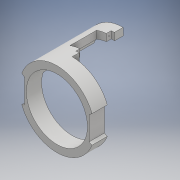
# Autodesk Inventor part: X-axis-gimbal-part
Saved by Autodesk Inventor 2017 (Build 210142000, 142)
## iProperties
Part Number: X-axis-gimbal-part
Material: 常规
Document SubType Name: Modeling
Designer: Lenovo
Density: 1 g/cm^3
Appearance: 默认
Author: Lenovo
Autodesk Inventor part; units mm, degrees
ref_plane "YZ Plane" through (0, 0, 0) normal (1, 0, 0) x (0, 1, 0)
ref_plane "XZ Plane" through (0, 0, 0) normal (0, 1, 0) x (-1, 0, 0)
sketch "Sketch1" plane through (0, 0, 0) normal (0, 1, 0) x (-1, 0, 0)
  circle A0 centre (0, 0) radius 37.0055
  circle A1 centre (0, 0) radius 29.8875
  constraints: 2 centre point, 2 coincident
extrude "Extrusion1" add sketch "Sketch1" along normal blind 15 contours A0 | A1
sketch "Sketch2" plane through (0, 15, 0) normal (0, 1, 0) x (1, 0, 0)
  circle A0 centre (0, 0) radius 37.0055 projected
  circle A1 centre (0, 0) radius 30.0306
  constraints: 1 centre point, 1 coincident
extrude "Extrusion2" cut sketch "Sketch2" against normal blind 15 contours A1
sketch "Sketch3" plane through (0, 15, 0) normal (0, 1, 0) x (1, 0, 0)
  circle A0 centre (0, 0) radius 37.0055 projected
  line L0 (-34.4949, -13.3982) -> (-31.6379, -11.0586)
  line L1 (-31.6379, -11.0586) -> (-31.6379, 12.0839)
  line L2 (-31.6379, 12.0839) -> (-34.4949, 13.3982)
  constraints: 6 end point, 2 point on circle, 1 vertical
extrude "Extrusion3" cut sketch "Sketch3" against normal blind 15 contours L2 L1 L0 A0 picked at (-33.4271, 0.3418)
sketch "Sketch4" plane through (0, 15, 0) normal (0, 1, 0) x (1, 0, 0)
  arc A0 (-34.4949, -13.3982) -> (-34.4949, 13.3982) centre (0, 0) ccw projected
  line L0 (-31.6379, -11.0586) -> (-31.6379, 12.0839) projected
  line L1 (31.575, 12.0839) -> (31.575, -11.0586)
  line L2 (31.575, -11.0586) -> (34.4949, -13.3982)
  line L3 (31.575, 12.0839) -> (34.4949, 13.3982)
  constraints: 6 end point, 2 point on circle
extrude "Extrusion4" cut sketch "Sketch4" against normal blind 15
sketch "Sketch5" plane through (0, 15, 0) normal (0, 1, 0) x (1, 0, 0)
  circle A0 centre (0, 0) radius 30.0306 projected
  line L0 (-31.6379, -11.0586) -> (-34.4949, -13.3982) projected
  arc A1 (-34.4949, -13.3982) -> (34.4949, -13.3982) centre (0, 0) ccw projected
  line L1 (-31.6379, -11.0586) -> (-31.6379, 12.0839) projected
  circle A2 centre (0, 0) radius 30.0306 projected
  line L2 (-31.6379, -11.0586) -> (-28.482, -9.519)
  line L3 (0, -37.0055) -> (0.2981, -30.0291)
  constraints: 5 point on circle, 4 end point
extrude "Extrusion5" add sketch "Sketch5" along normal blind 50 contours A0 L3 A1 L0 L2
ref_plane "Work Plane1" through (0, 15, 37.0055) normal (0, 0, 1) x (1, 0, 0)
sketch "Sketch6" plane through (0, 15, 37.0055) normal (0, 0, 1) x (1, 0, 0)
  line L0 (0.2981, 0) -> (0.2981, 50) projected
  line L1 (0.2981, 41.3903) -> (-3.1652, 41.3903)
  line L2 (-3.1652, 41.3903) -> (-3.1652, 36.7258)
  line L3 (-3.1652, 36.7258) -> (-12.8273, 36.7258)
  line L4 (-12.8273, 36.7258) -> (-12.8273, 10.738)
  line L5 (-12.8273, 10.738) -> (-3.1652, 10.738)
  line L6 (-3.1652, 10.738) -> (-3.1652, 6.7398)
  line L7 (-3.1652, 6.7398) -> (0.2981, 6.7398)
  point P0 (0, -15)
  constraints: 14 end point, 5 perpendicular, 2 horizontal, 2 point on line
extrude "Extrusion6" cut sketch "Sketch6" against normal blind 10
hole "Hole1" at (-3.1652, 23.7389, 33.3666) direction (-1, 0, 0) diameter 1 depth 3 tip angle 118
hole "Hole2" at (-3.1652, 54.058, 33.3666) direction (-1, 0, 0) diameter 1 depth 3 tip angle 118
body "Solid1"
